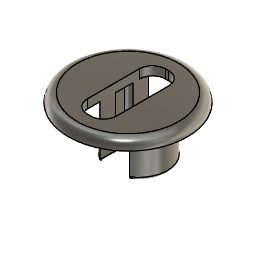
SNES - USB Cover v21 (Autodesk Fusion 360 design; units mm, degrees)
Autodesk Fusion 360 part; units mm, degrees
sketch "Boceto1" plane through (0, 0, 0) normal (0, 0, 1) x (1, 0, 0)
  line L0 (-1.675, 3.2) -> (1.675, 3.2)
  line L1 (1.675, 3.2) -> (1.675, -5.7)
  line L2 (1.675, -5.7) -> (-1.675, -5.7)
  line L3 (-1.675, -5.7) -> (-1.675, 3.2)
  circle A0 centre (0, -1.25) radius 6.75
  dimension "d16" = 3.35
  dimension "d17" = 1.675
  dimension "d18" = 5.7
  dimension "d27" = 3.2
  dimension "d33" = 13.5
  constraint horizontal L0
  constraint vertical L1
  constraint horizontal L2
  constraint vertical L3
  measures "d16" distance of L0.start L0.end
  measures "d17" horizontal distance of origin L0.start
  measures "d18" vertical distance of origin L2.end
  measures "d27" vertical distance of origin L0.start
  measures "d33" diameter of A0
extrude "Extruir1" add sketch "Boceto1" against normal blind 1
sketch "Boceto2" plane through (0, 0, -1) normal (0, 0, -1) x (1, 0, 0)
  line L0 (-1.675, 5.7) -> (1.675, 5.7)
  line L1 (1.675, 5.7) -> (1.675, -3.2)
  line L2 (1.675, -3.2) -> (-1.675, -3.2)
  line L3 (-1.675, -3.2) -> (-1.675, 5.7)
  circle A0 centre (0, 1.25) radius 6.75
  line L4 (1.675, -2.7559) -> (1.675, 2.7559)
  line L5 (-1.675, -2.7559) -> (-1.675, 2.7559)
  arc A1 (1.675, -2.7559) -> (1.675, 2.7559) centre (0, 0) ccw
  arc A2 (-1.675, 2.7559) -> (-1.675, -2.7559) centre (0, 0) ccw
  dimension "d38" = 6.45
  constraint coincident A1.centre A2.centre
  constraint coincident L1 L4.start
  constraint coincident L1 L4.end
  constraint coincident L3 L5.start
  constraint coincident L5.end A1
  constraint coincident L3 L5.end
  constraint concentric A1 A2
  measures "d38" diameter of A1
extrude "Extruir2" add sketch "Boceto1" against normal blind 6 contours L0 L1 L2 L3
extrude "Extruir3" cut sketch "Boceto1" against normal blind 10 contours L0 L1 L2 L3
fillet "Empalme2" radius 1.5 2 edges at (1.675, -5.7, -0.5) (-1.675, -5.7, -0.5)
fillet "Empalme2" radius 1.5 2 edges at (-1.675, 3.2, -0.5) (1.675, 3.2, -0.5)
fillet "Empalme4" radius 1 1 edges at (-6.2932, -3.6909, 0)
extrude "Extruir6" add sketch "Boceto2" along normal blind 6 contours L3 L5 A2 | L1 L4 A1
sketch "Boceto3" plane through (-1.675, 0, 0) normal (1, 0, 0) x (0, 1, 0)
  line L0 (2.7559, -7) -> (2.7559, -1)
  line L1 (2.7559, -1) -> (1.7, -1)
  line L2 (1.7, -1) -> (1.7, 0)
  line L3 (1.7, 0) -> (-4.2, 0)
  line L4 (-4.2, 0) -> (-4.2, -1)
  line L5 (-4.2, -1) -> (-2.7559, -1)
  line L6 (-2.7559, -1) -> (-2.7559, -7)
  line L7 (-2.7559, -7) -> (2.7559, -7)
  line L8 (1, -1) -> (1, -7)
  line L9 (-1, -1) -> (-1, -7)
  line L10 (1, -1) -> (-1, -1)
  dimension "d45" = 5.5118
  dimension "d46" = 1.7559
  dimension "d47" = 1.7559
  constraint coincident L7 L8.end
  constraint perpendicular L7 L8
  constraint coincident L7 L9.end
  constraint perpendicular L7 L9
  measures "d45" distance of L0 L6
  measures "d46" distance of L0 L8
  measures "d47" distance of L6 L9.end
extrude "Extruir7" cut sketch "Boceto3" against normal blind 0.5 contours L7 L8 L9 L10
sketch "Boceto4" plane through (1.675, 0, 0) normal (-1, 0, 0) x (0, -1, 0)
  line L0 (-1.7, 0) -> (-1.7, -1)
  line L1 (-1.7, -1) -> (-2.7559, -1)
  line L2 (-2.7559, -1) -> (-2.7559, -7)
  line L3 (-2.7559, -7) -> (2.7559, -7)
  line L4 (2.7559, -7) -> (2.7559, -1)
  line L5 (2.7559, -1) -> (4.2, -1)
  line L6 (4.2, -1) -> (4.2, 0)
  line L7 (4.2, 0) -> (-1.7, 0)
  line L8 (1, -7) -> (1, -1)
  line L9 (-1, -7) -> (-1, -1)
  line L10 (-1, -1) -> (1, -1)
  dimension "d50" = 1.7559
  dimension "d51" = 1.7559
  constraint coincident L3 L8.start
  constraint perpendicular L7 L8
  constraint coincident L3 L9.start
  constraint perpendicular L7 L9
  measures "d50" distance of L4 L8
  measures "d51" distance of L2 L9
extrude "Extruir8" cut sketch "Boceto4" against normal blind 0.5 contours L3 L8 L9 L10
fillet "Empalme5" radius 0.3 6 edges at (-3.225, 0, -7) (3.225, 0, -7) (1.675, 1.878, -7) (1.675, -1.878, -7) (-1.675, -1.878, -7) (-1.675, 1.878, -7)
fillet "Empalme6" radius 0.5 6 edges at (2.175, -1, -4) (2.175, 0, -1) (2.175, 1, -4) (-2.175, 1, -4) (-2.175, 0, -1) (-2.175, -1, -4)
equation "d1 = 6.4 mm"
equation "d2 = d1 + ( ( 2 * 1 ) * 1 mm )"
equation "d17 = d16 / 2"
equation "d46 = d45 / 2 - 1 mm"
equation "d47 = d45 / 2 - 1 mm"
equation "d50 = d45 / 2 - 1 mm"
equation "d51 = d45 / 2 - 1 mm"
